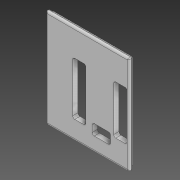
# Autodesk Inventor part: TAPA CASE UFOX
Saved by Autodesk Inventor 2021 (Build 250183000, 183)
## iProperties
Created: 2022-08-19
Part Number: TAPA CASE UFOX
Material: Genérico
Document SubType Name: Modeling
Designer: PC
Density: 1 g/cm^3
Appearance: Valor por defecto
Author: PC
Autodesk Inventor part; units mm, degrees
ref_plane "YZ Plane" through (0, 0, 0) normal (1, 0, 0) x (0, 1, 0)
ref_plane "XZ Plane" through (0, 0, 0) normal (0, 1, 0) x (-1, 0, 0)
ref_plane "XY Plane" through (0, 0, 0) normal (0, 0, 1) x (1, 0, 0)
sketch "Boceto1" plane through (0, 0, 0) normal (0, 0, 1) x (1, 0, 0)
  arc A0 (40.3152, 49.166) -> (39.3152, 50.166) centre (39.3152, 49.166) ccw
  line L0 (39.3152, 50.166) -> (-39.4848, 50.166)
  arc A1 (-39.4848, 50.166) -> (-40.4848, 49.166) centre (-39.4848, 49.166) ccw
  line L1 (-40.4848, 49.166) -> (-40.4848, -44.234)
  arc A2 (-40.4848, -44.234) -> (-39.4848, -45.234) centre (-39.4848, -44.234) ccw
  line L2 (-39.4848, -45.234) -> (39.3152, -45.234)
  arc A3 (39.3152, -45.234) -> (40.3152, -44.234) centre (39.3152, -44.234) ccw
  line L3 (40.3152, -44.234) -> (40.3152, 49.166)
  line L4 (38.8152, 47.666) -> (38.8152, -42.734)
  arc A4 (37.8152, -43.734) -> (38.8152, -42.734) centre (37.8152, -42.734) ccw
  line L5 (37.8152, -43.734) -> (-37.9848, -43.734)
  arc A5 (-38.9848, -42.734) -> (-37.9848, -43.734) centre (-37.9848, -42.734) ccw
  line L6 (-38.9848, -42.734) -> (-38.9848, 47.666)
  arc A6 (-37.9848, 48.666) -> (-38.9848, 47.666) centre (-37.9848, 47.666) ccw
  line L7 (-37.9848, 48.666) -> (37.8152, 48.666)
  arc A7 (38.8152, 47.666) -> (37.8152, 48.666) centre (37.8152, 47.666) ccw
  line L8 (37.8152, 48.316) -> (-37.9848, 48.316)
  arc A8 (-37.9848, 48.316) -> (-38.6348, 47.666) centre (-37.9848, 47.666) ccw
  line L9 (-38.6348, 47.666) -> (-38.6348, -42.734)
  arc A9 (-38.6348, -42.734) -> (-37.9848, -43.384) centre (-37.9848, -42.734) ccw
  line L10 (-37.9848, -43.384) -> (37.8152, -43.384)
  arc A10 (37.8152, -43.384) -> (38.4652, -42.734) centre (37.8152, -42.734) ccw
  line L11 (38.4652, -42.734) -> (38.4652, 47.666)
  arc A11 (38.4652, 47.666) -> (37.8152, 48.316) centre (37.8152, 47.666) ccw
  point P0 (0, 0)
  point P1 (0, 0)
  dimension "d0" = 0.35
  constraints: 24 end point, 24 point on circle, 12 centre point, 7 other
  measures "d0" distance between parallel lines of L7 L8
extrude "Extrusión1" add sketch "Boceto1" against normal blind 5 contours A11 L11 A10 L10 A9 L9 A8 L8
extrude "Extrusión2" add sketch "Boceto1" against normal blind 2.5 contours L3 A3 L2 A2 L1 A1 L0 A0 | L4 A4 L5 A5 L6 A6 L7 A7
sketch "Boceto2" plane through (0, 0, 0) normal (0, 0, 1) x (1, 0, 0)
  line L0 (-14.2913, 24.2197) -> (-10.2913, 24.2197)
  line L1 (-10.2913, 24.2197) -> (-10.2913, -26.972)
  line L2 (-10.2913, -26.972) -> (-14.2913, -26.972)
  line L3 (-14.2913, -26.972) -> (-14.2913, 24.2197)
  line L4 (-9.6113, 18.1347) -> (-1.5458, 18.1347)
  line L5 (-1.5458, 18.1347) -> (-1.5458, 2.4011)
  line L6 (-1.5458, 2.4011) -> (-9.6113, 2.4011)
  line L7 (-9.6113, 2.4011) -> (-9.6113, 18.1347)
  line L8 (34.3514, 24.2197) -> (38.3514, 24.2197)
  line L9 (38.3514, 24.2197) -> (38.3514, -14.8735)
  line L10 (38.3514, -14.8735) -> (34.3514, -14.8735)
  line L11 (34.3514, -14.8735) -> (34.3514, 24.2197)
  line L12 (25.4392, 22.8389) -> (31.2901, 22.8389)
  line L13 (31.2901, 22.8389) -> (31.2901, 6.3553)
  line L14 (31.2901, 6.3553) -> (25.4392, 6.3553)
  line L15 (25.4392, 6.3553) -> (25.4392, 22.8389)
  line L16 (25.4392, -5.1596) -> (31.2901, -5.1596)
  line L17 (31.2901, -5.1596) -> (31.2901, -17.8285)
  line L18 (31.2901, -17.8285) -> (25.4392, -17.8285)
  line L19 (25.4392, -17.8285) -> (25.4392, -5.1596)
  line L20 (31.2901, -18.4179) -> (37.2447, -18.4179)
  line L21 (37.2447, -18.4179) -> (37.2447, -22.8222)
  line L22 (37.2447, -22.8222) -> (31.2901, -22.8222)
  line L23 (31.2901, -22.8222) -> (31.2901, -18.4179)
  line L24 (-40.089, 47.3619) -> (-40.089, -46.0381)
  line L25 (38.3514, -22.8222) -> (25.4392, -22.8222)
  line L26 (25.4392, -22.8222) -> (25.4392, 24.2197)
  line L27 (25.4392, 24.2197) -> (38.3514, 24.2197)
  line L28 (38.3514, 24.2197) -> (38.3514, -22.8222)
  line L29 (-14.2913, -26.972) -> (-1.5458, -26.972)
  line L30 (-1.5458, -26.972) -> (-1.5458, 24.2197)
  line L31 (-1.5458, 24.2197) -> (-14.2913, 24.2197)
  line L32 (-14.2913, 24.2197) -> (-14.2913, -26.972)
  point P0 (0, 0)
  point P1 (-10.2913, -26.972)
  dimension "d5" = 4
  dimension "d6" = 4
  dimension "d7" = 25.7977
  dimension "d8" = 0.68
  dimension "d9" = 26.9851
  dimension "d10" = 3.0614
  dimension "d11" = 3.5444
  constraints: 66 end point, 16 parallel, 8 horizontal, 8 perpendicular, 3 collinear, 3 point on line
  measures "d5" distance between parallel lines of L3 L1
  measures "d6" distance between parallel lines of L11 L9
  measures "d7" distance between parallel lines of L24 L3
  measures "d8" distance between parallel lines of L7 L1
  measures "d9" distance between parallel lines of L15 L5
  measures "d10" distance between parallel lines of L13 L11
  measures "d11" distance between parallel lines of L10 L20
extrude "Extrusión3" cut sketch "Boceto2" against normal blind 5
sketch "Boceto3" plane through (0, 0, 0) normal (0, 0, 1) x (1, 0, 0)
  line L0 (4.6221, -21.0738) -> (22.2739, -21.0738)
  line L1 (22.2739, -21.0738) -> (22.2739, -31.4813)
  line L2 (22.2739, -31.4813) -> (4.6221, -31.4813)
  line L3 (4.6221, -31.4813) -> (4.6221, -21.0738)
  line L4 (-1.5822, 24.0639) -> (-1.5822, -27.1278)
  line L5 (25.4029, -22.978) -> (25.4029, 24.0639)
  point P0 (0, 0)
  point P1 (-0.1072, -19.9018)
  point P2 (78.8, -95.4)
  dimension "d14" = 6.2043
  dimension "d15" = 3.129
  dimension "d16" = 10.4074
  constraints: 12 end point, 2 parallel, 1 horizontal, 1 perpendicular
  measures "d14" distance between parallel lines of L4 L3
  measures "d15" distance between parallel lines of L5 L1
  measures "d16" distance between parallel lines of L2 L0
extrude "Extrusión4" cut sketch "Boceto3" against normal blind 5
fillet "Empalme1" radius 2 12 edges at (-14.2913, 24.2197, -2.5) (-1.5458, 24.2197, -2.5) (-1.5458, -26.972, -2.5) (-14.2913, -26.972, -2.5) (4.6221, -31.4813, -2.5) (4.6221, -21.0738, -2.5) (22.2739, -21.0738, -2.5) (22.2739, -31.4813, -2.5) (38.3514, -22.8222, -2.5) (25.4392, -22.8222, -2.5) (25.4392, 24.2197, -2.5) (38.3514, 24.2197, -2.5)
fillet "Empalme2" radius 2 8 edges at (-40.1919, 49.8731, 0) (-40.4848, 2.466, 0) (-40.1919, -44.9411, 0) (-0.0848, -45.234, 0) (40.0223, -44.9411, 0) (40.3152, 2.466, 0) (40.0223, 49.8731, 0) (-0.0848, 50.166, 0)
